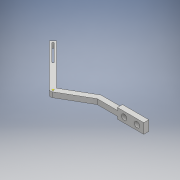
# Autodesk Inventor part: Ramię♥
Saved by Autodesk Inventor 2017 (Build 210142000, 142)
## iProperties
Created: 2018-05-29
Part Number: Ramię♥
Material: Generic
Document SubType Name: Modeling
Designer: Pies
Density: 1 g/cm^3
Appearance: Default
Author: Pies
Autodesk Inventor part; units mm, degrees
ref_plane "YZ Plane" through (0, 0, 0) normal (1, 0, 0) x (0, 1, 0)
ref_plane "XZ Plane" through (0, 0, 0) normal (0, 1, 0) x (-1, 0, 0)
ref_plane "XY Plane" through (0, 0, 0) normal (0, 0, 1) x (1, 0, 0)
sketch "Sketch1" plane through (0, 0, 0) normal (0, 0, 1) x (1, 0, 0)
  line L0 (37.3205, 11.5) -> (16.9186, 11.5)
  line L1 (-26.163, 24.0416) -> (-1.0607, -1.0607)
  line L2 (17.7224, 8.5) -> (0.75, -1.299)
  line L3 (17.7224, 8.5) -> (37.3205, 8.5)
  line L4 (0.2468, 1.8745) -> (16.9186, 11.5)
  line L5 (0.2468, 1.8745) -> (-24.0416, 26.163)
  arc A0 (-23.6881, 24.3952) -> (-24.3952, 23.6881) centre (-24.0416, 24.0416) ccw
  arc A1 (-14.4957, 13.7886) -> (-13.7886, 14.4957) centre (-14.1421, 14.1421) ccw
  circle A2 centre (0, 0) radius 0.5
  line L6 (-25.1023, 25.1023) -> (-26.163, 24.0416)
  line L7 (-24.0416, 26.163) -> (-25.1023, 25.1023)
  line L8 (-24.3952, 23.6881) -> (-14.4957, 13.7886)
  line L9 (-13.7886, 14.4957) -> (-23.6881, 24.3952)
  line L10 (37.3205, 8.5) -> (45.3205, 8.5)
  line L11 (45.3205, 8.5) -> (45.3205, 11.5)
  line L12 (45.3205, 11.5) -> (37.3205, 11.5)
  arc A3 (-1.0607, -1.0607) -> (0.75, -1.299) centre (0, 0) ccw
  constraints: 26 end point, 6 point on circle, 4 centre point, 3 parallel, 3 perpendicular, 2 coincident, 1 collinear, 1 horizontal, 1 point on line, 1 tangent
extrude "Extrusion1" add sketch "Sketch1" along normal blind 3
sketch "Sketch5" plane through (0, 0, 3) normal (0, 0, 1) x (1, 0, 0)
  point P0 (0, 0)
sketch "Sketch8" plane through (45.3205, 8.5, 0) normal (1, 0, 0) x (0, 0, -1)
  line L0 (0, 0) -> (-3, 0) projected
  line L1 (-3, 0) -> (-4.5, 0)
  line L2 (-4.5, 0) -> (-4.5, 3)
  line L3 (-4.5, 3) -> (1.5, 3)
  line L4 (1.5, 3) -> (1.5, 0)
  line L5 (1.5, 0) -> (-3, 0)
  point P0 (0, -8.5)
  dimension "d38" = 1.5
  dimension "d39" = 3
  dimension "d40" = 6
  dimension "d41" = 3
  constraints: 10 end point, 2 perpendicular, 1 collinear, 1 horizontal, 1 point on line
  measures "d38" distance of L0.end L1.end
  measures "d39" distance of L1.end L2.end
  measures "d40" distance of L2.end L3.end
  measures "d41" distance of L3.end L4.end
extrude "Extrusion4" add sketch "Sketch8" against normal blind 15.588
sketch "Sketch9" plane through (16.9186, 11.5, 3) normal (0, 1, 0) x (1, 0, 0)
  line L0 (28.4019, 4.5) -> (28.4019, -1.5) construction
  point P0 (-16.9186, 3)
  point P1 (24.4019, 1.5)
  point P2 (16.8139, 1.5)
hole "Hole2" at (41.3205, 11.5, 1.5) at (33.7325, 11.5, 1.5) direction (0, -1, 0) diameter 3.2 end through all clearance for "Hex Head Cap Screw ISO 24017" size "M3" standard "ISO"
body "Solid1"
